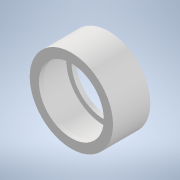
# Autodesk Inventor part: inner part
Saved by Autodesk Inventor 2021 (Build 250183000, 183)
## iProperties
Created: 2022-06-28
Part Number: inner part
Material: Типовые
Document SubType Name: Modeling
Designer: termi
Density: 1 g/cm^3
Appearance: По умолчанию
Author: termi
Autodesk Inventor part; units mm, degrees
ref_plane "YZ Plane" through (0, 0, 0) normal (1, 0, 0) x (0, 1, 0)
ref_plane "XZ Plane" through (0, 0, 0) normal (0, 1, 0) x (-1, 0, 0)
ref_plane "XY Plane" through (0, 0, 0) normal (0, 0, 1) x (1, 0, 0)
sketch "Эскиз1" plane through (0, 0, 0) normal (0, 1, 0) x (-1, 0, 0)
  line L0 (-5, -52) -> (-5, -72)
  line L1 (-145, -72) -> (-5, -72) projected
  line L2 (-5, 11) -> (-145, 11) projected
  line L3 (-5, -9) -> (-5, 11)
  line L4 (5, -0.6) -> (5, -2.7)
  line L5 (4.4, -61) -> (-154.4, -61) projected
  line L6 (-4.5, -61) -> (-4.5, -71)
  line L7 (-4.5, -71) -> (15.5, -71)
  line L8 (15.5, -71) -> (15.5, 10)
  line L9 (15.5, 10) -> (-4.5, 10)
  line L10 (-4.5, 10) -> (-4.5, 0)
  line L11 (-4.5, 0) -> (7, 0)
  line L12 (7, 0) -> (7, -61)
  line L13 (7, -61) -> (-4.5, -61)
  line L14 (-145, -9) -> (-145, 11)
  line L15 (-5, 11) -> (-145, 11) construction
  line L16 (-75, 11) -> (-75, -72)
  point P0 (0, 0)
  dimension "d0" = 10
  dimension "d1" = 20
  dimension "d2" = 0.5
  dimension "d3" = 0.5
  dimension "d4" = 10
  dimension "d5" = 2
  constraints: 28 end point, 7 perpendicular, 4 vertical, 2 collinear, 2 midpoint, 2 point on line, 6 other
  measures "d0" distance of L6.start L6.end
  measures "d1" distance of L6.end L7.end
  measures "d2" distance between parallel lines of L0 L6
  measures "d3" distance between parallel lines of L3 L10
  measures "d4" distance between parallel lines of L11 L9
  measures "d5" distance between parallel lines of L12 L4
revolve "Вращение1" add sketch "Эскиз1" angle 360 about axis through (75, 0, 11) along (0, 0, -1) contours L13 L12 L11 L10 L9 L8 L7 L6 L5
